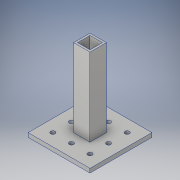
# Autodesk Inventor part: SupportPlateWithPostOnlyV01
Saved by Autodesk Inventor 2017 (Build 210142000, 142)
## iProperties
Created: 2016-02-07
Part Number: SupportPlateWithPostOnlyV01
Material: Aluminum 6061
Document SubType Name: Modeling
Designer: steele
Density: 2.7 g/cm^3
Appearance: Aluminum - Flat
Author: steele
Autodesk Inventor part; units mm, degrees
ref_plane "YZ Plane" through (0, 0, 0) normal (1, 0, 0) x (0, 1, 0)
ref_plane "XZ Plane" through (0, 0, 0) normal (0, 1, 0) x (-1, 0, 0)
ref_plane "XY Plane" through (0, 0, 0) normal (0, 0, 1) x (1, 0, 0)
sketch "Sketch1" plane through (0, 0, 0) normal (0, 1, 0) x (-1, 0, 0)
  line L0 (47.625, 47.625) -> (-47.625, 47.625)
  line L1 (-47.625, 47.625) -> (-47.625, -47.625)
  line L2 (-47.625, -47.625) -> (47.625, -47.625)
  line L3 (47.625, -47.625) -> (47.625, 47.625)
  line L4 (47.625, 47.625) -> (-47.625, -47.625) construction
  line L5 (-47.625, 47.625) -> (47.625, -47.625) construction
  point P0 (0, 0)
  dimension "d0" = 95.25
  dimension "d1" = 95.25
  constraints: 12 end point, 2 midpoint, 2 parallel, 1 horizontal, 1 perpendicular
  measures "d0" distance of L2.end L0.start
  measures "d1" distance of L0.start L0.end
extrude "Extrusion1" add sketch "Sketch1" along normal blind 6.35
sketch "Sketch2" plane through (0, 6.35, 0) normal (0, 1, 0) x (1, 0, 0)
  line L0 (-12.7, -12.7) -> (12.7, -12.7)
  line L1 (12.7, -12.7) -> (12.7, 12.7)
  line L2 (12.7, 12.7) -> (-12.7, 12.7)
  line L3 (-12.7, 12.7) -> (-12.7, -12.7)
  line L4 (-12.7, -12.7) -> (12.7, 12.7) construction
  line L5 (12.7, -12.7) -> (-12.7, 12.7) construction
  line L6 (-9.525, -9.525) -> (9.525, -9.525)
  line L7 (9.525, -9.525) -> (9.525, 9.525)
  line L8 (9.525, 9.525) -> (-9.525, 9.525)
  line L9 (-9.525, 9.525) -> (-9.525, -9.525)
  line L10 (-9.525, -9.525) -> (9.525, 9.525) construction
  line L11 (9.525, -9.525) -> (-9.525, 9.525) construction
  line L12 (47.625, -47.625) -> (47.625, 47.625) projected
  line L13 (-47.625, -47.625) -> (47.625, -47.625) projected
  point P0 (0, 0)
  point P1 (0, 0)
  dimension "d4" = 25.4
  dimension "d5" = 25.4
  dimension "d6" = 3.175
  dimension "d7" = 3.175
  dimension "d8" = 34.925
  dimension "d14" = 34.925
  constraints: 24 end point, 4 midpoint, 4 parallel, 2 horizontal, 2 perpendicular
  measures "d4" distance of L0.end L1.end
  measures "d5" distance of L1.end L2.end
  measures "d6" distance between parallel lines of L6 L0
  measures "d7" distance between parallel lines of L9 L3
  measures "d8" distance between parallel lines of L1 L12
  measures "d14" distance between parallel lines of L0 L13
extrude "Extrusion2" add sketch "Sketch2" along normal blind 119.9388
sketch "Sketch12" plane through (0, 6.35, 0) normal (0, 1, 0) x (1, 0, 0)
  line L0 (-28.575, -28.575) -> (34.925, -28.575) construction
  line L1 (-28.575, -28.575) -> (-28.575, 34.925) construction
  line L2 (-47.625, -47.625) -> (47.625, -47.625) construction
  circle A0 centre (-28.575, -28.575) radius 3.3782
  circle A1 centre (0, -28.575) radius 3.3782
  circle A2 centre (28.575, -28.575) radius 3.3782
  circle A3 centre (-28.575, 0) radius 3.3782
  circle A4 centre (0, 0) radius 3.3782
  circle A5 centre (28.575, 0) radius 3.3782
  circle A6 centre (-28.575, 28.575) radius 3.3782
  circle A7 centre (0, 28.575) radius 3.3782
  circle A8 centre (28.575, 28.575) radius 3.3782
  point P0 (0, 0)
  dimension "d52" = 19.05
  dimension "d53" = 19.05
  dimension "d57" = 6.7564
  dimension "d60" = 28.575
  dimension "d63" = 28.575
  constraints: 9 centre point, 4 end point, 2 horizontal, 2 vertical, 1 coincident, 16 other
  measures "d52" distance between parallel lines of L0 L2
  measures "d53" distance from line of L2.start L1
  measures "d57" diameter of A0
  measures "d60" distance of A0.centre A1.centre
  measures "d63" distance of A0.centre A3.centre
extrude "Extrusion8" cut sketch "Sketch12" against normal blind 25.4
sketch "Sketch8" plane through (-12.7, 6.35, 12.7) normal (0, 0, 1) x (1, 0, 0)
  point P0 (12.7, 50.8)
sketch "Sketch9" plane through (-9.525, 6.35, -9.525) normal (0, 0, 1) x (1, 0, 0)
  point P0 (9.525, 50.8)
equation "\"d0\" = width"
equation "\"d1\" = length"
equation "\"d2\" = thickness"
equation "\"d9\" = heightOfPostAbovePlate"
equation "\"width\" = 95.25"
equation "\"length\" = 95.25"
equation "\"thickness\" = 6.35"
equation "\"totalHeight\" = 152.4"
equation "\"distanceFromFloorToBottomOfPan\" = 26.1112"
equation "\"thicknessOfPan\" = 3.175"
equation "\"heightOfPostAbovePlate\" = -thickness + totalHeight - distanceFromFloorToBottomOfPan"
body "Solid1"
